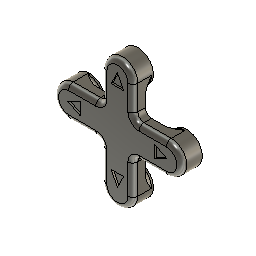
D-Pad DC32 v3 (Autodesk Fusion 360 design; units mm, degrees)
Autodesk Fusion 360 part; units mm, degrees
sketch "Sketch1" plane through (0, 0, 0) normal (0, 1, 0) x (1, 0, 0)
  line L0 (-20.3998, 2.605) -> (-4.5998, 2.605)
  line L1 (-4.5998, 2.605) -> (-4.5998, -2.395)
  line L2 (-4.5998, -2.395) -> (-20.3998, -2.395)
  line L3 (-20.3998, -2.395) -> (-20.3998, 2.605)
  line L4 (-20.3998, -2.395) -> (-4.5998, 2.605) construction
  line L5 (-20.3998, 2.605) -> (-4.5998, -2.395) construction
  line L6 (-12.4998, 0.105) -> (-12.4998, -7.395) construction
  line L7 (-9.9998, -7.395) -> (-14.9998, -7.395)
  line L8 (-14.9998, -7.395) -> (-14.9998, 8.405)
  line L9 (-14.9998, 8.405) -> (-9.9998, 8.405)
  line L10 (-9.9998, 8.405) -> (-9.9998, -7.395)
  line L11 (-12.4998, 0.105) -> (-12.4998, 8.405) construction
  line L12 (-12.4998, 0.105) -> (-4.5998, 0.105) construction
  line L13 (-12.4998, 0.105) -> (-20.2712, 0.105) construction
  circle A0 centre (-4.5998, 0.105) radius 2.5
  circle A1 centre (-12.4998, -7.395) radius 2.5
  circle A2 centre (-20.2712, 0.105) radius 2.5033
  circle A3 centre (-12.4998, 8.405) radius 2.5
  dimension "d3" = 15.8
  dimension "d8" = 15.8
  dimension "d47" = 5
  dimension "d48" = 5
  constraint horizontal L0
  constraint vertical L1
  constraint horizontal L2
  constraint vertical L3
  constraint midpoint L4 L6.start
  constraint perpendicular L2 L6
  constraint horizontal L7
  constraint vertical L8
  constraint horizontal L9
  constraint vertical L10
  constraint midpoint L9 L11.end
  constraint perpendicular L9 L11
  constraint midpoint L1 L12.end
  constraint perpendicular L3 L13
  constraint coincident L12.end A0.centre
  constraint coincident L1.end A0
  constraint coincident L6.end A1.centre
  constraint coincident L7.start A1
  constraint tangent L10 A1
  constraint coincident L13.end A2.centre
  constraint coincident L2.end A2
  constraint coincident L11.end A3.centre
  constraint coincident L9.end A3
  measures "d3" distance of L1 L3
  measures "d8" distance of L7.start L9.end
  measures "d47" distance of L8.end L9.end
  measures "d48" distance of L0.start L2.end
extrude "Extrude1" add sketch "Sketch1" along normal blind 2 contours L0 L2 L3 A2 | L3 A2 | L0 L2 L8 A2 | L0 L8 L10 A3 | L0 L2 L8 L10 | L0 L2 L10 A0 | L2 L8 L10 A1 | L9 A3 | L9 A3 | L1 A0 | L1 A0 | L7 A1 | L7 A1
sketch "Sketch2" plane through (0, 2, 0) normal (0, 1, 0) x (-1, 0, 0)
  line L0 (20.3998, 2.395) -> (14.9998, 2.395)
  line L1 (14.9998, 2.395) -> (14.9998, 7.395)
  line L2 (9.9998, 7.395) -> (9.9998, 2.395)
  line L3 (9.9998, 2.395) -> (4.5998, 2.395)
  line L4 (4.5998, -2.605) -> (9.9998, -2.605)
  arc A0 (4.5998, 2.395) -> (4.5998, -2.605) centre (4.5998, -0.105) ccw
  arc A1 (20.3998, -2.605) -> (20.3998, 2.395) centre (20.2712, -0.105) ccw
  arc A2 (14.9998, 7.395) -> (9.9998, 7.395) centre (12.4998, 7.395) ccw
  line L5 (9.9998, -2.605) -> (9.9998, -8.405)
  arc A3 (9.9998, -8.405) -> (14.9998, -8.405) centre (12.4998, -8.405) ccw
  line L6 (14.9998, -8.405) -> (14.9998, -2.605)
  line L7 (14.9998, -2.605) -> (20.3998, -2.605)
  circle A4 centre (12.4998, 7.395) radius 1.15
  circle A5 centre (20.2712, -0.105) radius 1.15
  circle A6 centre (4.5998, -0.105) radius 1.15
  circle A7 centre (12.4998, -8.405) radius 1.15
  circle A8 centre (20.2712, -0.105) radius 2.5033
  circle A9 centre (12.4998, 7.395) radius 2.5
  circle A10 centre (4.5998, -0.105) radius 2.5
  circle A11 centre (12.4998, -8.405) radius 2.5
  dimension "d50" = 2.3
  dimension "d51" = 2.3
  dimension "d52" = 2.3
  dimension "d53" = 2.3
  constraint concentric A2 A4
  constraint concentric A1 A5
  constraint concentric A0 A6
  constraint concentric A3 A7
  constraint concentric A1 A8
  constraint coincident A1.start A8
  constraint concentric A4 A9
  constraint coincident L1.end A9
  constraint concentric A0 A10
  constraint coincident L3.end A10
  constraint concentric A7 A11
  constraint coincident L5.end A11
  measures "d50" diameter of A4
  measures "d51" diameter of A5
  measures "d52" diameter of A6
  measures "d53" diameter of A7
extrude "Extrude2" add sketch "Sketch2" along normal blind 1.3 contours L0 A1 L7 A8 | A2 A9 | A3 A11 | A0 A10
sketch "Sketch3" plane through (0, 0, 0) normal (0, -1, 0) x (1, 0, 0)
  line L0 (-12.5, 7.5) -> (-12.5, 8)
  line L1 (-12.5, 8) -> (-12.5, 7.5)
  line L2 (-12.5, 7.5) -> (-12.5, 6)
  line L3 (-12.5, 6) -> (-11.5, 6)
  line L4 (-12.5, 6) -> (-13.5, 6)
  line L5 (-13.5, 6) -> (-12.5, 8)
  line L6 (-11.5, 6) -> (-12.5, 8)
  line L7 (-10.6998, 1.695) -> (-14.2998, -1.8) construction
  line L8 (-14.2998, 1.695) -> (-20.3998, -2.605) construction
  line L9 (-20, 0) -> (-20.5, 0)
  line L10 (-20, 0) -> (-18.5, 0)
  line L11 (-18.5, 0) -> (-18.5, 1)
  line L12 (-18.5, 0) -> (-18.5, -1)
  line L13 (-20.5, 0) -> (-18.5, 1)
  line L14 (-18.5, -1) -> (-20.5, 0)
  line L15 (-5, 0) -> (-4.5, 0)
  line L16 (-5, 0) -> (-6.5, 0)
  line L17 (-6.5, 0) -> (-6.5, 1)
  line L18 (-6.5, 0) -> (-6.5, -1)
  line L19 (-6.5, 1) -> (-4.5, 0)
  line L20 (-6.5, -1) -> (-4.5, 0)
  line L21 (-12.5, -7.5) -> (-12.5, -8)
  line L22 (-12.5, -8) -> (-12.5, -7.5)
  line L23 (-12.5, -7.5) -> (-12.5, -6)
  line L24 (-12.5, -6) -> (-11.5, -6)
  line L25 (-12.5, -6) -> (-13.5, -6)
  line L26 (-13.5, -6) -> (-12.5, -8)
  line L27 (-11.5, -6) -> (-12.5, -8)
  arc A0 (-20.3998, 2.395) -> (-20.3998, -2.605) centre (-20.2712, -0.105) ccw
  line L28 (-9.9998, -8.405) -> (-9.9998, -2.605)
  line L29 (-9.9998, -2.605) -> (-4.5998, -2.605)
  arc A1 (-4.5998, -2.605) -> (-4.5998, 2.395) centre (-4.5998, -0.105) ccw
  line L30 (-4.5998, 2.395) -> (-9.9998, 2.395)
  line L31 (-9.9998, 2.395) -> (-9.9998, 7.395)
  arc A2 (-9.9998, 7.395) -> (-14.9998, 7.395) centre (-12.4998, 7.395) ccw
  line L32 (-14.9998, 7.395) -> (-14.9998, 2.395)
  line L33 (-14.9998, 2.395) -> (-20.3998, 2.395)
  line L34 (-20.3998, -2.605) -> (-14.9998, -2.605)
  line L35 (-14.9998, -2.605) -> (-14.9998, -8.405)
  arc A3 (-14.9998, -8.405) -> (-9.9998, -8.405) centre (-12.4998, -8.405) ccw
  dimension "d31" = 1.5
  dimension "d32" = 1
  dimension "d33" = 1
  dimension "d34" = 0.5
  dimension "d35" = 1.5
  dimension "d36" = 1
  dimension "d37" = 1
  dimension "d38" = 0.5
  dimension "d39" = 1.5
  dimension "d40" = 1
  dimension "d41" = 1
  dimension "d42" = 1.5
  dimension "d43" = 1
  dimension "d44" = 1
  constraint vertical L0
  constraint parallel L0 L1
  constraint parallel L0 L2
  constraint perpendicular L2 L3
  constraint perpendicular L2 L4
  constraint coincident L8.end A0.end
  constraint parallel L9 L10
  constraint perpendicular L10 L11
  constraint perpendicular L10 L12
  constraint parallel L15 L16
  constraint perpendicular L16 L17
  constraint perpendicular L16 L18
  constraint perpendicular L23 L24
  constraint perpendicular L23 L25
  measures "d31" distance of L0.start L2.end
  measures "d32" distance of L2.end L3.end
  measures "d33" distance of L2.end L4.end
  measures "d34" distance of L9.start L9.end
  measures "d35" distance of L9.start L10.end
  measures "d36" distance of L10.end L11.end
  measures "d37" distance of L10.end L12.end
  measures "d38" distance of L15.start L15.end
  measures "d39" distance of L15.start L16.end
  measures "d40" distance of L16.end L17.end
  measures "d41" distance of L16.end L18.end
  measures "d42" distance of L21.start L23.end
  measures "d43" distance of L23.end L24.end
  measures "d44" distance of L23.end L25.end
extrude "Extrude3" cut sketch "Sketch3" against normal blind 0.3 contours L0 L1 L2 L4 L5 | L0 L1 L2 L3 L6 | L9 L10 L12 L14 | L9 L10 L11 L13 | L15 L16 L17 L19 | L15 L16 L18 L20 | L21 L22 L23 L24 L27 | L21 L22 L23 L25 L26
fillet "Fillet4" radius 1 4 edges at (-17.7679, 2, -0.105) (-12.4998, 2, -5.905) (-12.4998, 2, 4.895) (-7.0998, 2, -0.105)
fillet "Fillet5" radius 1 4 edges at (-9.9998, 1, 2.395) (-14.9998, 1, 2.395) (-14.9998, 1, -2.605) (-9.9998, 1, -2.605)
fillet "Fillet7" radius 0.8 16 edges at (-18.1998, 0, -2.605) (-15.2927, 0, -2.8979) (-14.9998, 0, -6.005) (-12.4998, 0, -10.905) (-9.9998, 0, -6.005) (-9.7069, 0, -2.8979) (-6.7998, 0, -2.605) (-2.0998, 0, -0.105) (-6.7998, 0, 2.395) (-9.7069, 0, 2.6879) (-9.9998, 0, 5.395) (-12.4998, 0, 9.895) (-14.9998, 0, 5.395) (-15.2927, 0, 2.6879) (-18.1998, 0, 2.395) (-22.7745, 0, -0.105)
